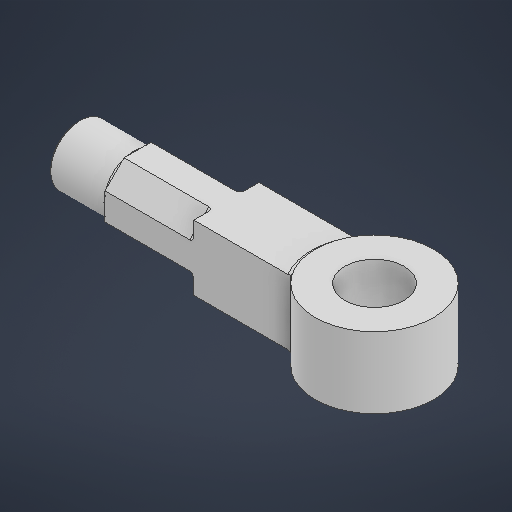
# Autodesk Inventor part: eye end
Saved by Autodesk Inventor 2026.3 (Build 303398000, 398)
## iProperties
Created: 2026-07-15
Part Number: eye end
Material: Generic
Document SubType Name: Modeling
Designer: User
Density: 1 g/cm^3
Appearance: Default
Author: User
Autodesk Inventor part; units mm, degrees
ref_plane "YZ Plane" through (0, 0, 0) normal (1, 0, 0) x (0, 1, 0)
ref_plane "XZ Plane" through (0, 0, 0) normal (0, 1, 0) x (-1, 0, 0)
ref_plane "XY Plane" through (0, 0, 0) normal (0, 0, 1) x (1, 0, 0)
sketch "Sketch1" plane through (0, 0, 0) normal (1, 0, 0) x (0, 1, 0)
  line L0 (16.5, 16.5) -> (-16.5, 16.5)
  line L1 (-16.5, 16.5) -> (-16.5, -16.5)
  line L2 (-16.5, -16.5) -> (16.5, -16.5)
  line L3 (16.5, -16.5) -> (16.5, 16.5)
  line L4 (16.5, 16.5) -> (-16.5, -16.5) construction
  line L5 (-16.5, 16.5) -> (16.5, -16.5) construction
  point P0 (0, 0)
  dimension "d0" = 33
  dimension "d1" = 33
  constraints: 12 end point, 2 midpoint, 2 parallel, 1 horizontal, 1 perpendicular
  measures "d0" distance of L2.end L1.end
  measures "d1" distance of L1.end L0.end
extrude "Extrusion1" add sketch "Sketch1" against normal blind 120
sketch "Sketch2" plane through (0, 0, 0) normal (0, 1, 0) x (-1, 0, 0)
  circle A0 centre (0, 0) radius 30
  dimension "d4" = 60
  constraints: 1 centre point, 1 coincident
  measures "d4" diameter of A0
extrude "Extrusion2" add sketch "Sketch2" along normal mid plane 36
sketch "Sketch3" plane through (0, 18, 0) normal (0, 1, 0) x (1, 0, 0)
  circle A0 centre (0, 0) radius 15
  dimension "d7" = 30
  constraints: 1 centre point, 1 coincident
  measures "d7" diameter of A0
extrude "Extrusion3" cut sketch "Sketch3" against normal through all
sketch "Sketch4" plane through (-120, 0, 0) normal (-1, 0, 0) x (0, 0, 1)
  line L0 (16.5, -16.5) -> (16.5, 16.5) projected
  line L1 (16.5, -6.8345) -> (6.8345, -16.5)
  line L2 (6.8345, -16.5) -> (-6.8345, -16.5)
  line L3 (-6.8345, -16.5) -> (-16.5, -6.8345)
  line L4 (-16.5, -6.8345) -> (-16.5, 6.8345)
  line L5 (-16.5, 6.8345) -> (-6.8345, 16.5)
  line L6 (-6.8345, 16.5) -> (6.8345, 16.5)
  line L7 (6.8345, 16.5) -> (16.5, 6.8345)
  line L8 (16.5, 6.8345) -> (16.5, -6.8345)
  line L9 (-16.5, -16.5) -> (16.5, -16.5) projected
  line L10 (16.5, -16.5) -> (16.5, 16.5) projected
  line L11 (16.5, 16.5) -> (-16.5, 16.5) projected
  line L12 (-16.5, 16.5) -> (-16.5, -16.5) projected
  point P0 (0, 0)
  point P1 (0, 0)
  point P2 (16.5, 0)
  constraints: 16 end point, 2 midpoint, 1 coincident, 17 other
extrude "Extrusion4" cut sketch "Sketch4" against normal blind 45 contours L9 L1 L0 | L7 L11 L0 | L9 L12 L3 | L5 L12 L11
sketch "Sketch5" plane through (-120, 0, 0) normal (-1, 0, 0) x (0, 0, 1)
  circle A0 centre (0, 0) radius 15
  dimension "d12" = 30
  constraints: 1 centre point, 1 coincident
  measures "d12" diameter of A0
extrude "Extrusion5" add sketch "Sketch5" along normal blind 30
fillet "Fillet1" radius 2 11 edges at (-25.0549, 0, 16.5) (-75, 11.6673, 11.6673) (-75, -11.6673, 11.6673) (-75, -11.6673, -11.6673) (-75, 11.6673, -11.6673) (-25.0549, 0, -16.5) (-28.7372, 16.5, 8.6125) (-28.7372, 16.5, -8.6125) (-28.7372, -16.5, -8.6125) (-28.7372, -16.5, 8.6125) (-120, 0, -15)
chamfer "Chamfer1" distance 1 angle 45 1 edges at (-150, 0, -15)
body "Solid1"
